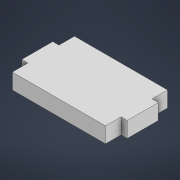
# Autodesk Inventor part: Подставка для двигателя и драйвера
Saved by Autodesk Inventor 2022 (Build 260153000, 153)
## iProperties
Created: 2023-02-18
Part Number: Подставка для двигателя и драйвера
Material: Типовые
Document SubType Name: Modeling
Designer: Глеб
Density: 1 g/cm^3
Appearance: По умолчанию
Author: Глеб
Autodesk Inventor part; units mm, degrees
ref_plane "YZ Plane" through (0, 0, 0) normal (1, 0, 0) x (0, 1, 0)
ref_plane "XZ Plane" through (0, 0, 0) normal (0, 1, 0) x (-1, 0, 0)
ref_plane "XY Plane" through (0, 0, 0) normal (0, 0, 1) x (1, 0, 0)
sketch "Эскиз1" plane through (0, 0, 0) normal (1, 0, 0) x (0, 1, 0)
  line L0 (-5, 10) -> (5, 10)
  line L1 (5, 10) -> (5, -10)
  line L2 (5, -10) -> (-5, -10)
  line L3 (-5, -10) -> (-5, 10)
  line L4 (-5, 10) -> (5, -10) construction
  line L5 (5, 10) -> (-5, -10) construction
  point P0 (0, 0)
  dimension "d0" = 10
  dimension "d1" = 20
  constraints: 12 end point, 2 midpoint, 2 parallel, 1 horizontal, 1 perpendicular
  measures "d0" distance between parallel lines of L3 L1
  measures "d1" distance between parallel lines of L2 L0
extrude "Выдавливание1" add sketch "Эскиз1" along normal mid plane 68
sketch "Эскиз2" plane through (-34, 5, 10) normal (0, 1, 0) x (1, 0, 0)
  line L0 (0, 20) -> (68, 20) projected
  line L1 (4, 20) -> (64, 20)
  line L2 (64, 20) -> (64, 30)
  line L3 (64, 30) -> (4, 30)
  line L4 (4, 30) -> (4, 20)
  line L5 (0, 0) -> (68, 0) projected
  line L6 (34, 20) -> (34, 0) construction
  line L7 (4, -10) -> (64, -10)
  line L8 (64, -10) -> (64, 0)
  line L9 (64, 0) -> (4, 0)
  line L10 (4, 0) -> (4, -10)
  line L11 (0, 0) -> (0, 20) projected
  line L12 (68, 20) -> (68, 0) projected
  point P0 (34, 10)
  point P1 (35, -10)
  point P2 (64, 0)
  point P3 (4, 0)
  dimension "d4" = 60
  dimension "d5" = 10
  dimension "d7" = 60
  dimension "d8" = 10
  dimension "d11" = 4
  constraints: 18 end point, 4 parallel, 2 horizontal, 2 midpoint, 2 perpendicular, 2 point on line, 1 collinear, 1 other
  measures "d4" distance of L2.end L3.end
  measures "d5" distance of L1.end L2.end
  measures "d7" distance of L8.end L9.end
  measures "d8" distance of L7.end L8.end
  measures "d11" distance between parallel lines of L11 L10
extrude "Выдавливание2" add sketch "Эскиз2" against normal blind 10 contours L4 L3 L2 L0 | L5 L8 L7 L10
equation "\"d7\" = d4"
equation "\"d8\" = d5"
